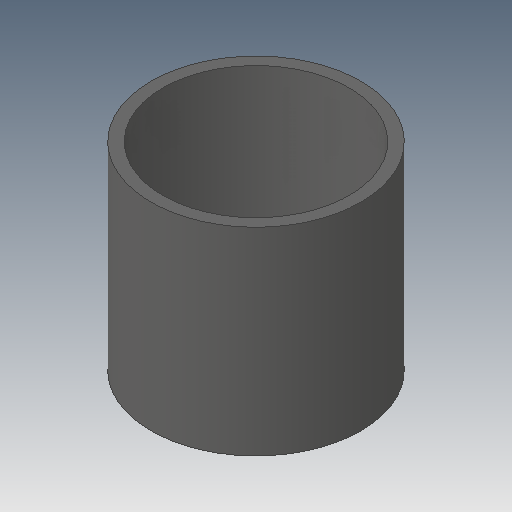
# Autodesk Inventor part: RUBBER2
Saved by Autodesk Inventor 2019 (Build 230136000, 136)
## iProperties
Created: 2023-06-18
Part Number: RUBBER2
Material: Generic
Document SubType Name: Modeling
Designer: Fransic
Density: 1 g/cm^3
Appearance: Gray
Mass: 0.90792 g
Surface Area: 19.2265 cm^2
Volume: 0.90792 cm^3
Author: Fransic
Autodesk Inventor part; units mm, degrees
ref_plane "YZ Plane" through (0, 0, 0) normal (1, 0, 0) x (0, 1, 0)
ref_plane "XZ Plane" through (0, 0, 0) normal (0, 1, 0) x (-1, 0, 0)
ref_plane "XY Plane" through (0, 0, 0) normal (0, 0, 1) x (1, 0, 0)
sketch "Sketch1" plane through (0, 0, 0) normal (0, 1, 0) x (-1, 0, 0)
  circle A0 centre (0, 0) radius 9
  dimension "d0" = 18
  constraints: 1 centre point, 1 coincident
  measures "d0" diameter of A0
extrude "Extrusion1" add sketch "Sketch1" along normal blind 17
shell "Shell1" thickness 1 removed faces 2 at (-2.2455, 0, -1.9894) at (-2.2455, 17, -1.9894)
body "Solid1"
